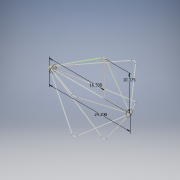
# Autodesk Inventor part: bicon_NateMeasurements
Saved by Autodesk Inventor 2019 (Build 230136000, 136)
## iProperties
Created: 2018-07-24
Part Number: bicon_NateMeasurements
Material: Generic
Document SubType Name: Modeling
Designer: User
Density: 1 g/cm^3
Appearance: Default
Author: User
Autodesk Inventor part; units mm, degrees
ref_plane "YZ Plane" through (0, 0, 0) normal (1, 0, 0) x (0, 1, 0)
ref_plane "XZ Plane" through (0, 0, 0) normal (0, 1, 0) x (-1, 0, 0)
ref_plane "XY Plane" through (0, 0, 0) normal (0, 0, 1) x (1, 0, 0)
sketch "Sketch1" plane through (0, 0, 0) normal (0, 0, 1) x (1, 0, 0)
  line L0 (614.68, 0) -> (0, 0) construction
  line L1 (0, 0) -> (400.0412, 259.793)
  line L2 (614.68, 0) -> (435.4312, 253.0151)
  line L3 (400.0412, 259.793) -> (420.9909, 273.3981) construction
  line L4 (435.4312, 253.0151) -> (420.9909, 273.3981) construction
  arc A0 (435.4312, 253.0151) -> (400.0412, 259.793) centre (414.2075, 237.9792) ccw
  line L5 (419.1, 0) -> (419.1, 263.525) construction
  dimension "d3" = 614.68
  dimension "d4" = 263.525
  dimension "d5" = 419.1
  constraints: 12 end point, 3 point on circle, 2 collinear, 1 centre point, 1 equal length, 1 horizontal, 1 perpendicular, 1 point on line, 1 tangent
  measures "d3" distance of L0.start L0.end
  measures "d4" distance of L5.start L5.end
  measures "d5" distance from line of L5 L0.end
ref_plane "Work Plane1" through (0, 0, 0) normal (0.8386675, 0.5446438, 0) x (-0.5446438, 0.8386675, 0)
sketch "Sketch2" plane through (0, 0, 0) normal (0.8386675, 0.5446438, 0) x (-0.5446438, 0.8386675, 0)
  circle A0 centre (0, 0) radius 3.175
  dimension "d0" = 6.35
  constraints: 1 centre point, 1 coincident
  measures "d0" diameter of A0
sweep "Sweep1" add profiles "Sketch2" path "Sketch1" path curves L1 A0 L2
pattern_circular "Circular Pattern1" count 6 over 360 about axis through (0, 0, 0) along (1, 0, 0) of "Sweep1"
sketch "Sketch3" plane through (0, 0, 0) normal (0, 0, 1) x (1, 0, 0)
  point P0 (0, 0)
sketch "Sketch5" plane through (0, 0, 0) normal (0, 0, 1) x (1, 0, 0)
  line L0 (-2.8092, 3.75) -> (32.1908, 26.4795)
  line L1 (32.1908, 26.4795) -> (32.1908, -26.4795)
  line L2 (32.1908, -26.4795) -> (-2.8092, -3.75) construction
  line L3 (-2.8092, -3.75) -> (-2.8092, 3.75)
  line L4 (-125.8951, 0) -> (741.1317, 0) projected
  line L5 (419.1, -87.5666) -> (419.1, 320.7928) projected
  line L6 (32.1908, 0) -> (-2.8092, 0)
  ellipse E0 centre (0, 0) end of major axis (10.2079, 4.8678) minor radius 2.8347 (5.8295, 0) -> (-1.5564, 2.3966) ccw projected
  ellipse E1 centre (0, 0) end of major axis (10.2079, 4.8678) minor radius 2.8347 (5.8295, 0) -> (-1.5564, 2.3966) ccw projected
  line L7 (-1.5564, 2.3966) -> (-1.5564, 2.3966) projected
  line L8 (401.7704, 257.1302) -> (398.312, 262.4558) projected
  line L9 (0, 0) -> (400.0412, 259.793) projected
  line L10 (12.5651, 8.16) -> (10.0189, 12.0807) construction
  line L11 (26.5946, 17.271) -> (24.0484, 21.1917) construction
  dimension "d11" = 35
  dimension "d24" = 4.675
  dimension "d25" = 7.5
  constraints: 14 end point, 6 point on line, 3 perpendicular, 2 midpoint, 2 parallel, 3 other
  measures "d11" distance between parallel lines of L1 L3
  measures "d24" distance of L10.start L10.end
  measures "d25" distance of L2.end L0.start
revolve "Revolution1" add sketch "Sketch5" angle 360 about axis through (0, 0, 0) along (1, 0, 0)
sketch "Sketch6" plane through (0, 0, 0) normal (0, 0, 1) x (1, 0, 0)
  line L0 (-128.9761, 0) -> (761.752, 0) projected
  line L1 (595.1881, 15.5) -> (595.1881, -15.5)
  line L2 (606.1881, 24) -> (606.1881, -24)
  line L3 (619.1881, 5) -> (619.1881, -5)
  line L4 (595.1881, 15.5) -> (606.1881, 24)
  line L5 (619.1881, 5) -> (606.1881, 24)
  line L6 (595.1881, -15.5) -> (606.1881, -24) construction
  line L7 (606.1881, -24) -> (619.1881, -5) construction
  line L8 (614.68, 0) -> (435.4312, 253.0151) projected
  line L9 (595.1881, 0) -> (619.1881, 0)
  point P0 (0, 0)
  point P1 (600.6881, 19.75)
  dimension "d26" = 31
  dimension "d27" = 48
  dimension "d28" = 10
  dimension "d29" = 13
  dimension "d30" = 24
  constraints: 16 end point, 3 midpoint, 2 equal length, 2 parallel, 1 perpendicular, 1 point on line, 1 other
  measures "d26" distance of L1.start L1.end
  measures "d27" distance of L2.start L2.end
  measures "d28" distance of L3.start L3.end
  measures "d29" distance between parallel lines of L3 L2
  measures "d30" distance between parallel lines of L3 L1
revolve "Revolution2" add sketch "Sketch6" angle 360 about axis through (0, 0, 0) along (1, 0, 0)
sketch "Sketch7" plane through (32.1908, 0, 0) normal (1, 0, 0) x (0, 0, -1)
  circle A0 centre (0, 0) radius 3.175
  point P0 (0, 0)
  dimension "d18" = 6.35
  constraints: 1 centre point, 1 coincident
  measures "d18" diameter of A0
extrude "Extrusion1" add sketch "Sketch7" along normal up to next
sketch "Sketch8" plane through (0, 0, 0) normal (0, 1, 0) x (-1, 0, 0)
  circle A0 centre (-419.1, 0) radius 3.175
  point P0 (0, 0)
  dimension "d21" = 6.35
  constraints: 1 centre point, 1 coincident
  measures "d21" diameter of A0
extrude "Extrusion2" add sketch "Sketch8" along normal up to next
body "Solid1"
